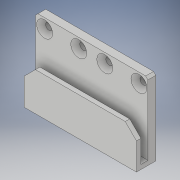
# Autodesk Inventor part: HX711MountingBracketv2
Saved by Autodesk Inventor 2019.3 (Build 233278000, 278)
## iProperties
Created: 2019-02-16
Part Number: HX711MountingBracketv2
Material: Generic
Document SubType Name: Modeling
Designer: mark
Density: 1 g/cm^3
Appearance: Default
Author: mark
Autodesk Inventor part; units mm, degrees
ref_plane "YZ Plane" through (0, 0, 0) normal (1, 0, 0) x (0, 1, 0)
ref_plane "XZ Plane" through (0, 0, 0) normal (0, 1, 0) x (-1, 0, 0)
ref_plane "XY Plane" through (0, 0, 0) normal (0, 0, 1) x (1, 0, 0)
sketch "Sketch1" plane through (0, 0, 0) normal (0, 0, 1) x (1, 0, 0)
  line L0 (0, 0) -> (50, 0)
  line L1 (50, 0) -> (50, 34)
  line L2 (50, 34) -> (0, 34)
  line L3 (0, 34) -> (0, 0)
  circle A0 centre (4, 29.625) radius 1.55
  circle A1 centre (19.2, 29.625) radius 1.55
  circle A2 centre (30.8, 29.625) radius 1.55
  circle A3 centre (46, 29.625) radius 1.55
  dimension "d0" = 50
  dimension "d1" = 34
  dimension "d2" = 4.375
  dimension "d3" = 4.375
  dimension "d4" = 4.375
  dimension "d5" = 4.375
  dimension "d6" = 15.2
  dimension "d7" = 15.2
  dimension "d8" = 34
  dimension "d9" = 4
  dimension "d10" = 4
  dimension "d11" = 3.1
  dimension "d12" = 3.1
  dimension "d13" = 3.1
  dimension "d14" = 3.1
  constraints: 8 end point, 4 centre point, 1 horizontal
  measures "d0" distance between parallel lines of L1 L3
  measures "d1" distance between parallel lines of L0 L2
  measures "d2" distance from line of L2 A0.centre
  measures "d3" distance from line of L2 A1.centre
  measures "d4" distance from line of A2.centre L2
  measures "d5" distance from line of L2 A3.centre
  measures "d6" distance of A3.centre A2.centre
  measures "d7" distance of A1.centre A0.centre
  measures "d8" distance of L2.end L0.start
  measures "d9" distance from line of L3 A0.centre
  measures "d10" distance from line of L1 A3.centre
  measures "d11" diameter of A0
  measures "d12" diameter of A1
  measures "d13" diameter of A2
  measures "d14" diameter of A3
extrude "Extrusion1" add sketch "Sketch1" along normal blind 3.5
sketch "Sketch2" plane through (0, 0, 3.5) normal (0, 0, 1) x (1, 0, 0)
  line L0 (0, 2) -> (50, 2)
  line L1 (50, 2) -> (50, 0)
  line L2 (50, 0) -> (0, 0)
  line L3 (0, 0) -> (0, 2)
  line L4 (0, 0) -> (50, 0) projected
  line L5 (0, 34) -> (0, 0) projected
  line L6 (50, 0) -> (50, 34) projected
  dimension "d17" = 2
  constraints: 8 end point, 3 collinear
  measures "d17" distance between parallel lines of L2 L0
extrude "Extrusion2" add sketch "Sketch2" along normal blind 5.1
sketch "Sketch3" plane through (0, 2, 3.5) normal (0, 1, 0) x (1, 0, 0)
  line L0 (0, -5.1) -> (50, -5.1)
  line L1 (50, -5.1) -> (50, -3.1)
  line L2 (50, -3.1) -> (0, -3.1)
  line L3 (0, -3.1) -> (0, -5.1)
  line L4 (0, 0) -> (0, -5.1) projected
  line L5 (50, 0) -> (50, -5.1) projected
  line L6 (50, -5.1) -> (0, -5.1) projected
  line L7 (50, 0) -> (0, 0) projected
  point P0 (0, 3.5)
  dimension "d20" = 3.1
  constraints: 8 end point, 3 collinear
  measures "d20" distance between parallel lines of L2 L7
extrude "Extrusion3" add sketch "Sketch3" along normal blind 15 contours L3 L2 L1 L0
chamfer "Chamfer1" distance 5 angle 45 2 edges at (50, 17, 7.6) (0, 17, 7.6)
chamfer "Chamfer2" distance 2 angle 45 4 edges at (2.45, 29.625, 3.5) (17.65, 29.625, 3.5) (29.25, 29.625, 3.5) (44.45, 29.625, 3.5)
chamfer "Chamfer3" distance 1 angle 45 2 edges at (0, 34, 1.75) (50, 34, 1.75)
body "Solid1"
